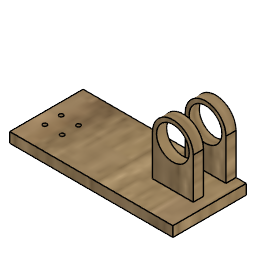
Base (Autodesk Fusion 360 design; units mm, degrees)
Autodesk Fusion 360 part; units mm, degrees
note: some values were not read from the file. Set by a fixed rule: which sketch regions a step uses; the direction of a hole.
sketch "Sketch1" plane through (0, 0, 0) normal (0, 0, 1) x (1, 0, 0)
  line L0 (0, 0) -> (20, 0)
  line L1 (20, 0) -> (20, 11)
  line L2 (20, 11) -> (0, 11)
  line L3 (0, 11) -> (0, 0)
  line L4 (0, 0) -> (80, 0)
  line L5 (0, 11) -> (0, 26)
  line L6 (0, 26) -> (80, 26)
  line L7 (80, 26) -> (80, 0)
  line L8 (80, 0) -> (0, 0)
  line L9 (0, 0) -> (0, 26)
  line L10 (80, 0) -> (80, -10)
  line L11 (80, -10) -> (0, -10)
  line L12 (0, -10) -> (0, 0)
  point P0 (5.75, 9.5)
  point P1 (14.25, 9.5)
  point P2 (14.25, 1.5)
  point P3 (5.75, 1.5)
  dimension "d1" = 20
  dimension "d2" = 11
  dimension "d3" = 1.5
  dimension "d4" = 1.5
  dimension "d5" = 8.5
  dimension "d6" = 5.75
  dimension "d7" = 80
  dimension "d8" = 15
  dimension "d19" = 10
  constraint horizontal L0
  constraint vertical L1
  constraint horizontal L2
  constraint vertical L3
  constraint coincident L0.start L3.end
  constraint horizontal P0 P1
  constraint horizontal P2 P3
  constraint vertical P1 P2
  constraint vertical P0 P3
  constraint perpendicular L3 L4
  constraint perpendicular L2 L5
  constraint horizontal L6
  constraint vertical L7
  constraint horizontal L8
  constraint vertical L9
  constraint vertical L10
  constraint horizontal L11
  constraint vertical L12
  constraint coincident L4.end L7.end
  measures "d1" distance of L0.start L0.end
  measures "d2" distance of L0.start L2.end
  measures "d3" distance of L2 P0
  measures "d4" distance of L0 P3
  measures "d5" distance of P0 P1
  measures "d6" distance of L3 P0
  measures "d7" distance of L0.start L4.end
  measures "d8" distance of L2.end L5.end
  measures "d19" distance of L0.start L11.end
extrude "Extrude1" add sketch "Sketch1" along normal blind 5
hole "Hole1" at (14.25, 1.5, 0) direction (0, 0, 1) diameter 2 end through all
pattern_linear "R-Pattern1" count 2 spacing 8.5 along (-1, 0, 0) count 2 spacing 8 along (0, 1, 0) of "Hole1"
sketch "Sketch2" plane through (0, 26, 0) normal (0, 1, 0) x (-1, 0, 0)
  line L0 (-80, 0) -> (0, 0)
  line L1 (0, 0) -> (0, 5)
  line L2 (0, 5) -> (-80, 5)
  line L3 (-80, 5) -> (-80, 0)
  circle A0 centre (-65, 25) radius 8
  line L4 (-73, 25) -> (-73, 5)
  line L5 (-57, 25) -> (-57, 5)
  line L6 (-57, 5) -> (-73, 5)
  circle A1 centre (-65, 25) radius 10
  line L7 (-75, 25) -> (-75, 5)
  line L8 (-55, 25) -> (-55, 5)
  dimension "d24" = 16
  dimension "d25" = 7
  dimension "d27" = 20
  dimension "d28" = 2
  dimension "d29" = 2
  dimension "d30" = -2
  constraint coincident A0 L4.start
  constraint coincident L2 L4.end
  constraint perpendicular L2 L4
  constraint coincident A0 L5.start
  constraint coincident L2 L5.end
  constraint perpendicular L2 L5
  constraint horizontal A0.centre L4.start
  constraint horizontal A0.centre L5.start
  measures "d24" diameter of A0
  measures "d25" distance of L2.end L4.end
  measures "d27" distance of A0.centre L6
extrude "Extrude2" add sketch "Sketch2" against normal blind 5 contours L2 L4 A1 L7 | L2 L5 A1 L8 | L2 L4 L5 L6 A1 | A0 L4 L5 A1 | A0 L4 L5 A1
ref_plane "WorkPlane2" through (65, 15.5, 20) normal (0, -1, 0) x (1, 0, 0)
mirror "Mirror1" about plane through (65, 15.5, 20) normal (0, -1, 0) of "Extrude2"
equation "d33 = ( 11 / 2 ) * 1 mm"
